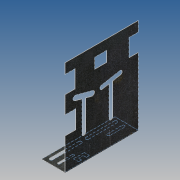
# Autodesk Inventor part: Platina lateral interna 2
Saved by Autodesk Inventor 2016 (Build 200138000, 138)
## iProperties
Created: 2016-05-25
Part Number: Platina lateral interna 2
Material: Steel
Document SubType Name: Modeling
Designer: Familia
Density: 7.85 g/cm^3
Appearance: Plate
Mass: 53.2474 g
Surface Area: 277.865 cm^2
Volume: 6.78311 cm^3
Author: Familia
Autodesk Inventor part; units mm, degrees
ref_plane "YZ Plane" through (0, 0, 0) normal (1, 0, 0) x (0, 1, 0)
ref_plane "XZ Plane" through (0, 0, 0) normal (0, 1, 0) x (-1, 0, 0)
ref_plane "XY Plane" through (0, 0, 0) normal (0, 0, 1) x (1, 0, 0)
sketch "Sketch1" plane through (0, 0, 0) normal (0, 1, 0) x (-1, 0, 0)
  line L0 (0, 0) -> (0, 130)
  line L1 (0, 130) -> (0.5, 130)
  line L2 (0.5, 130) -> (0.5, 0.5)
  line L3 (0.5, 0.5) -> (32, 0.5)
  line L4 (32, 0.5) -> (32, 0)
  line L5 (32, 0) -> (0, 0)
  dimension "d0" = 0.5
  dimension "d1" = 130
  dimension "d2" = 32
  constraints: 12 end point, 6 perpendicular, 1 vertical
  measures "d0" distance of L0.end L1.end
  measures "d1" distance of L0.start L0.end
  measures "d2" distance between parallel lines of L4 L0
extrude "Extrusion1" add sketch "Sketch1" along normal mid plane 100
sketch "Sketch2" plane through (0, -50, 0) normal (1, 0, 0) x (0, 0, -1)
  line L0 (-116.2978, 40.4754) -> (-102.0897, 40.4754)
  line L1 (-102.0897, 40.4754) -> (-102.0897, 56.9569)
  line L2 (-102.0897, 56.9569) -> (-116.2978, 56.9569)
  line L3 (-116.2978, 56.9569) -> (-116.2978, 40.4754)
  line L4 (-116.2978, -0.6285) -> (-92.269, -0.6285)
  line L5 (-92.269, -0.6285) -> (-92.269, 13.8246)
  line L6 (-92.269, 13.8246) -> (-116.2978, 13.8246)
  line L7 (-116.2978, 13.8246) -> (-116.2978, -0.6285)
  line L8 (-68.5175, -0.6285) -> (-43.5049, -0.6285)
  line L9 (-43.5049, -0.6285) -> (-43.5049, 14.8755)
  line L10 (-43.5049, 14.8755) -> (-68.5175, 14.8755)
  line L11 (-68.5175, 14.8755) -> (-68.5175, -0.6285)
  line L12 (-116.2978, 101.3011) -> (-92.269, 101.3011)
  line L13 (-92.269, 101.3011) -> (-92.269, 87.6013)
  line L14 (-92.269, 87.6013) -> (-116.2978, 87.6013)
  line L15 (-116.2978, 87.6013) -> (-116.2978, 101.3011)
  line L16 (-33.7527, 25.6785) -> (-78.3542, 25.6785) construction
  line L17 (-33.7527, 23.1785) -> (-78.3542, 23.1785)
  line L18 (-78.3542, 28.1785) -> (-33.7527, 28.1785)
  arc A0 (-33.7527, 23.1785) -> (-33.7527, 28.1785) centre (-33.7527, 25.6785) ccw
  arc A1 (-78.3542, 28.1785) -> (-78.3542, 23.1785) centre (-78.3542, 25.6785) ccw
  line L19 (-33.7526, 62.8674) -> (-78.3542, 62.8674) construction
  line L20 (-33.7526, 65.3674) -> (-78.3542, 65.3674)
  line L21 (-78.3542, 60.3674) -> (-33.7526, 60.3674)
  arc A2 (-33.7526, 60.3674) -> (-33.7526, 65.3674) centre (-33.7526, 62.8674) ccw
  arc A3 (-78.3542, 65.3674) -> (-78.3542, 60.3674) centre (-78.3542, 62.8674) ccw
  line L22 (-76.0973, 50.4436) -> (-80.6111, 75.2913) construction
  line L23 (-73.3501, 50.9427) -> (-77.8639, 75.7903)
  line L24 (-83.3583, 74.7922) -> (-78.8445, 49.9445)
  arc A4 (-78.8445, 49.9445) -> (-73.3501, 50.9427) centre (-76.0973, 50.4436) ccw
  arc A5 (-77.8639, 75.7903) -> (-83.3583, 74.7922) centre (-80.6111, 75.2913) ccw
  line L25 (-75.2925, 37.1839) -> (-81.416, 14.1731) construction
  line L26 (-78.3502, 37.9976) -> (-84.4737, 14.9868)
  line L27 (-78.3582, 13.3594) -> (-72.2347, 36.3702)
  arc A6 (-72.2347, 36.3702) -> (-78.3502, 37.9976) centre (-75.2925, 37.1839) ccw
  arc A7 (-84.4737, 14.9868) -> (-78.3582, 13.3594) centre (-81.416, 14.1731) ccw
  point P0 (0, 50)
  point P1 (-56.0534, 25.6785)
  point P2 (-56.0534, 62.8674)
  dimension "d16" = 2.5
  constraints: 64 end point, 16 point on circle, 16 tangent, 13 parallel, 8 centre point, 5 horizontal, 4 midpoint, 4 perpendicular, 3 point on line, 1 equal radius, 1 vertical alignment
  measures "d16" radius of A2
extrude "Extrusion2" cut sketch "Sketch2" against normal blind 100
sketch "Sketch5" plane through (-32, 50, 0.5) normal (0, 0, 1) x (1, 0, 0)
  line L0 (6.4118, -5.271) -> (6.4118, -44.3585) construction
  line L1 (4.397, -5.271) -> (4.397, -44.3585)
  line L2 (8.4266, -44.3585) -> (8.4266, -5.271)
  arc A0 (8.4266, -5.271) -> (4.397, -5.271) centre (6.4118, -5.271) ccw
  arc A1 (4.397, -44.3585) -> (8.4266, -44.3585) centre (6.4118, -44.3585) ccw
  line L3 (6.4118, -53.8282) -> (6.4118, -93.3186) construction
  line L4 (4.397, -53.8282) -> (4.397, -93.3186)
  line L5 (8.4266, -93.3186) -> (8.4266, -53.8282)
  arc A2 (8.4266, -53.8282) -> (4.397, -53.8282) centre (6.4118, -53.8282) ccw
  arc A3 (4.397, -93.3186) -> (8.4266, -93.3186) centre (6.4118, -93.3186) ccw
  line L6 (16.7722, -25.4192) -> (16.7722, -5.271) construction
  line L7 (14.9589, -25.4192) -> (14.9589, -5.271)
  line L8 (18.5856, -5.271) -> (18.5856, -25.4192)
  arc A4 (14.9589, -25.4192) -> (18.5856, -25.4192) centre (16.7722, -25.4192) ccw
  arc A5 (18.5856, -5.271) -> (14.9589, -5.271) centre (16.7722, -5.271) ccw
  line L9 (16.7722, -73.5734) -> (16.7722, -93.3186) construction
  line L10 (15.3955, -73.5734) -> (15.3955, -93.3186)
  line L11 (18.1489, -93.3186) -> (18.1489, -73.5734)
  arc A6 (18.1489, -73.5734) -> (15.3955, -73.5734) centre (16.7722, -73.5734) ccw
  arc A7 (15.3955, -93.3186) -> (18.1489, -93.3186) centre (16.7722, -93.3186) ccw
  line L12 (28.3587, -63.1068) -> (21.2143, -63.1068)
  line L13 (21.2143, -63.1068) -> (21.2143, -77.826)
  line L14 (21.2143, -77.826) -> (28.3587, -77.826)
  line L15 (28.3587, -77.826) -> (28.3587, -73.5734)
  line L16 (28.3587, -73.5734) -> (24.1409, -73.5734)
  line L17 (24.1409, -73.5734) -> (24.1409, -67.3246)
  line L18 (24.1409, -67.3246) -> (28.3587, -67.3246)
  line L19 (28.3587, -67.3246) -> (28.3587, -63.1068)
  point P0 (32, -50)
  point P1 (6.4118, -24.8148)
  point P2 (6.4118, -73.5734)
  point P3 (16.7722, -15.3451)
  point P4 (16.7722, -83.446)
  constraints: 49 end point, 16 point on circle, 16 tangent, 8 centre point, 6 perpendicular, 5 parallel, 4 midpoint, 4 point on line, 2 vertical, 1 horizontal
extrude "Extrusion5" cut sketch "Sketch5" against normal blind 10
body "Solid1"
